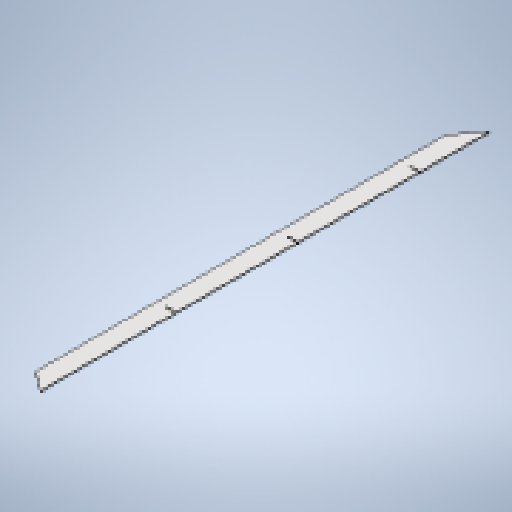
# Autodesk Inventor part: MSC 602 stringer cone exit back
Saved by Autodesk Inventor 2025 (Build 290162010, 162A)
## iProperties
Created: 2024-08-26
Part Number: MSC 602 stringer cone exit back
Material: Stainless Steel
Document SubType Name: Sheet Metal
Designer: pokla
Density: 8 g/cm^3
Sheet Metal Rule: AISI304 3mm Die 32
Appearance: Default
Stock Number: МОО 602 стрингер конус выход корма
Mass: 1359.31 g
Surface Area: 1209.85 cm^2
Volume: 169.914 cm^3
Flat Pattern Width: 5 cm
Flat Pattern Length: 118.581 cm
Flat Pattern Area: 592.903 cm^2
Sheet Metal Width: 50,000 mm
Sheet Metal Length: 1185,806 mm
Sheet Metal Area: 59290,309 mm^2
Author: pokla
Autodesk Inventor part; units mm, degrees
ref_plane "YZ Plane" through (0, 0, 0) normal (1, 0, 0) x (0, 1, 0)
ref_plane "XZ Plane" through (0, 0, 0) normal (0, 1, 0) x (-1, 0, 0)
ref_plane "XY Plane" through (0, 0, 0) normal (0, 0, 1) x (1, 0, 0)
sketch "Sketch1" plane through (0, 0, 0) normal (0, 0, 1) x (1, 0, 0)
  line L0 (-25, 0) -> (25, 0)
  line L1 (25, 0) -> (25, -1190)
  line L2 (25, -1190) -> (-25, -1190)
  line L3 (-25, -1190) -> (-25, 0)
  line L4 (25, -1190) -> (-25, -1153.2713)
  line L5 (25, 0) -> (-25, -68.0668)
  point P0 (0, 0)
  point P1 (0, 0)
  point P2 (25, -1153.2713)
  dimension "d0" = 50
  dimension "d1" = 1190
  dimension "d5" = 53.7
  dimension "d6" = 53.7
  measures "d0" distance of L0.start L0.end
  measures "d1" distance of L2.end L0.start
  measures "d5" angle of L4 L3
  measures "d6" angle of L0 L5
extrude "Plate1" add sketch "Sketch1" along normal mid plane 3 contours L1 L4 L3 L5
chamfer "Corner Chamfer1" distance 3 angle 45 1 edges at (25, -1190, 0)
fillet "Corner Round1" radius 6 1 edges at (-25, -1153.2713, 0)
fillet "Corner Round2" radius 6 1 edges at (-25, -68.0668, 0)
chamfer "Corner Chamfer3" distance 3 angle 45 1 edges at (25, 0, 0)
sketch "Sketch3" plane through (0, 0, 1.5) normal (0, 0, 1) x (1, 0, 0)
  line L0 (-1, -188.5) -> (25, -188.5)
  line L1 (25, -188.5) -> (25, -185.5)
  line L2 (25, -185.5) -> (-1, -185.5)
  line L3 (-1, -185.5) -> (-1, -188.5)
  line L4 (25, -3) -> (25, -1187) projected
  point P0 (0, 0)
  point P1 (25, -187)
  dimension "d18" = 187
  dimension "d19" = 26
  dimension "d20" = 3
  constraints: 8 end point, 2 parallel, 1 horizontal, 1 midpoint, 1 perpendicular, 1 point on line
  measures "d18" vertical distance of point (0, 0) point (25, -187)
  measures "d19" distance of L0.start L0.end
  measures "d20" distance of L2.end L0.start
extrude "Extrusion1" cut sketch "Sketch3" against normal through all
pattern_linear "Rectangular Pattern1" count 3 spacing 323 along (0, -1, 0) of "Extrusion1"
equation "\"d6\" = d5"
equation "\"d2\" = Thickness"
equation "\"BendReliefWidth\" = Thickness"
equation "\"BendReliefDepth\" = 0.5 * Thickness"
equation "\"CornerReliefSize\" = 4 * Thickness"
equation "\"MinimumRemnant\" = 2 * Thickness"
equation "\"TransitionRadius\" = BendRadius"
equation "\"JacobiRadiusSize\" = BendRadius"
equation "\"GapSize\" = Thickness"
equation "\"Thickness\" = 3"
equation "\"BendRadius\" = 5"
body "Solid1"
